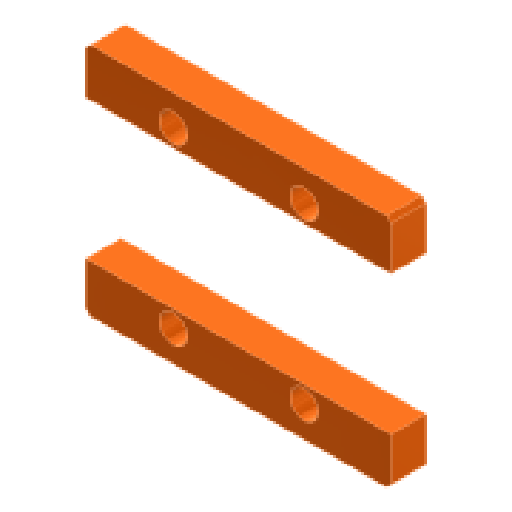
# Autodesk Inventor part: Gantry_Baseblock
Saved by Autodesk Inventor 2023.2 (Build 272271000, 271)
## iProperties
Created: 2023-02-03
Part Number: Gantry_Baseblock
Material: ABS Plastic
Document SubType Name: Modeling
Designer: remop
Density: 1.06 g/cm^3
Appearance: Smooth - Light Orange
Author: remop
Autodesk Inventor part; units mm, degrees
ref_plane "YZ Plane" through (0, 0, 0) normal (1, 0, 0) x (0, 1, 0)
ref_plane "XZ Plane" through (0, 0, 0) normal (0, 1, 0) x (-1, 0, 0)
ref_plane "XY Plane" through (0, 0, 0) normal (0, 0, 1) x (1, 0, 0)
sketch "Sketch2" plane through (0, 0, 0) normal (0, 0, 1) x (1, 0, 0)
  circle A0 centre (-7.5, 10) radius 1.6
  circle A1 centre (7.5, 10) radius 1.6
  circle A2 centre (7.5, -10) radius 1.6
  circle A3 centre (-7.5, -10) radius 1.6
  line L0 (-17.5, 8) -> (17.5, 8)
  line L1 (17.5, 8) -> (17.5, 13)
  line L2 (17.5, 13) -> (17, 13.5)
  line L3 (17, 13.5) -> (-17, 13.5)
  line L4 (-17, 13.5) -> (-17.5, 13)
  line L5 (-17.5, 13) -> (-17.5, 8)
  line L6 (-17.5, -8) -> (17.5, -8)
  line L7 (17.5, -8) -> (17.5, -13)
  line L8 (17.5, -13) -> (17, -13.5)
  line L9 (17, -13.5) -> (-17, -13.5)
  line L10 (-17, -13.5) -> (-17.5, -13)
  line L11 (-17.5, -13) -> (-17.5, -8)
  point P0 (0, 0)
  dimension "d3" = 15
  dimension "d4" = 20
  dimension "d5" = 3.2
  dimension "d6" = 7.5
  dimension "d7" = 2
  dimension "d8" = 10
  dimension "d9" = 10
  dimension "d10" = 3.5
  dimension "d11" = 45
  dimension "d12" = 5
  dimension "d13" = 10
  dimension "d16" = 2
  constraints: 24 end point, 8 equal length, 4 centre point, 3 equal radius, 3 parallel, 3 vertical alignment, 2 horizontal, 2 horizontal alignment, 2 perpendicular, 1 vertical
  measures "d3" distance of A1.centre A0.centre
  measures "d4" distance of A2.centre A1.centre
  measures "d5" diameter of A0
  measures "d6" horizontal distance of A1.centre point (0, 0)
  measures "d7" distance from line of L0 A0.centre
  measures "d8" distance from line of A0.centre L5
  measures "d9" distance from line of L1 A1.centre
  measures "d10" distance from line of A0.centre L3
  measures "d11" angle of L5 L4
  measures "d12" distance of L4.end L0.start
  measures "d13" vertical distance of A1.centre point (0, 0)
  measures "d16" distance from line of L6 A3.centre
extrude "Extrusion1" add sketch "Sketch2" along normal blind 4
equation "\"d6\" = 0.5 * d3"
equation "\"d9\" = d8"
equation "\"d13\" = 0.5 * d4"
equation "\"d16\" = d7"
body "Solid1"
